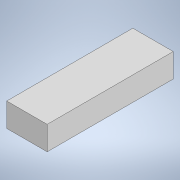
# Autodesk Inventor part: Accumulator-01
Saved by Autodesk Inventor 2020 (Build 240168000, 168)
## iProperties
Created: 2020-03-03
Part Number: Accumulator-01
Material: Generic
Document SubType Name: Modeling
Designer: valem
Density: 1 g/cm^3
Appearance: Default
Author: valem
Autodesk Inventor part; units mm, degrees
note: some values were not read from the file. Left out: dimensions or parameters whose unit could not be read.
ref_plane "YZ Plane" through (0, 0, 0) normal (1, 0, 0) x (0, 1, 0)
ref_plane "XZ Plane" through (0, 0, 0) normal (0, 1, 0) x (-1, 0, 0)
ref_plane "XY Plane" through (0, 0, 0) normal (0, 0, 1) x (1, 0, 0)
sketch "Sketch1" plane through (0, 0, 0) normal (0, 0, 1) x (1, 0, 0)
  line L0 (-17, 10) -> (17, 10)
  line L1 (17, 10) -> (17, -10)
  line L2 (17, -10) -> (-17, -10)
  line L3 (-17, -10) -> (-17, 10)
  line L4 (-17, -10) -> (17, 10) construction
  line L5 (-17, 10) -> (17, -10) construction
  point P0 (0, 0)
  point P1 (0, 0)
  point P2 (0, 0)
  dimension "d0" = 20
  dimension "d1" = 34
  constraints: 12 end point, 3 midpoint, 2 parallel, 1 coincident, 1 horizontal, 1 perpendicular
  measures "d0" distance of L0.end L1.end
  measures "d1" distance of L0.start L0.end
extrude "Extrusion1" add sketch "Sketch1" against normal blind 106
equation "\"d0\" = height"
equation "\"d1\" = width"
equation "\"d2\" = length"
equation "\"width\" = 34"
equation "\"height\" = 20"
equation "\"length\" = 106"
body "Solid1"
